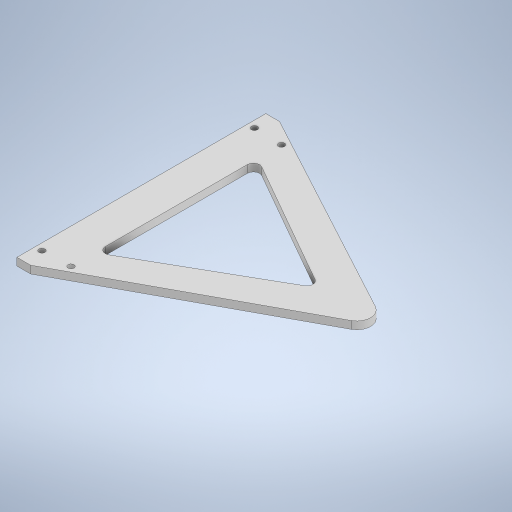
# Autodesk Inventor part: 17 nueva
Saved by Autodesk Inventor 2024.2 (Build 282272000, 272)
## iProperties
Created: 2024-10-10
Part Number: 17 nueva
Material: Generic
Document SubType Name: Modeling
Designer: Precisión-04
Density: 1 g/cm^3
Appearance: Default
Author: Precisión-04
Autodesk Inventor part; units mm, degrees
ref_plane "YZ Plane" through (0, 0, 0) normal (1, 0, 0) x (0, 1, 0)
ref_plane "XZ Plane" through (0, 0, 0) normal (0, 1, 0) x (-1, 0, 0)
ref_plane "XY Plane" through (0, 0, 0) normal (0, 0, 1) x (1, 0, 0)
sketch "Sketch1" plane through (0, 0, 0) normal (0, 1, 0) x (-1, 0, 0)
  line L0 (0, 0) -> (0, -164)
  line L1 (0, 0) -> (-9, 0)
  line L2 (0, -164) -> (-9, -164)
  line L3 (56.0828, -82) -> (-131.3763, -82) construction
  arc A0 (-146.3035, -74.0793) -> (-146.3035, -89.9207) centre (-142.03, -82) ccw
  line L4 (-110.9841, -85.4733) -> (-28.9841, -132.315)
  line L5 (-110.9833, -78.5263) -> (-28.9833, -31.7073)
  arc A1 (-23, -35.1809) -> (-28.9833, -31.7073) centre (-27, -35.1809) ccw
  arc A2 (-28.9841, -132.315) -> (-23, -128.8417) centre (-27, -128.8417) ccw
  line L6 (-23, -35.1809) -> (-23, -128.8417)
  line L7 (-146.3035, -89.9207) -> (-9, -164)
  line L8 (-9, 0) -> (-146.3035, -74.0793)
  arc A3 (-110.9833, -78.5263) -> (-110.9841, -85.4733) centre (-109, -82) ccw
  point P0 (0, -82)
  point P1 (-23, -82)
  point P2 (-75.5556, -35.9087)
  point P3 (-69.9833, -55.1168)
  point P4 (-75.5113, -128.1152)
  point P5 (-69.9841, -108.8941)
  dimension "d0" = 164
  dimension "d1" = 9
  dimension "d2" = 9
  dimension "d13" = 18
  dimension "d20" = 8
  dimension "d21" = 8
  dimension "d73" = 142.03
  dimension "d74" = 23
  dimension "d76" = 8
  dimension "d77" = 86
  dimension "d78" = 20
  dimension "d79" = 20
  constraints: 18 end point, 8 point on circle, 8 tangent, 7 point on line, 4 centre point, 3 horizontal, 3 midpoint, 2 vertical
  measures "d0" distance of L0.start L0.end
  measures "d1" distance of L0.start L1.end
  measures "d2" distance of L0.end L2.end
  measures "d13" diameter of A0
  measures "d20" diameter of A1
  measures "d21" diameter of A2
  measures "d73" distance from line of L0 A0.centre
  measures "d74" distance between parallel lines of L0 L6
  measures "d76" diameter of A3
  measures "d77" distance from line of L6 A3.centre
  measures "d78" distance of point (-75.556, -35.909) point (-69.983, -55.117)
  measures "d79" distance of point (-75.511, -128.115) point (-69.984, -108.894)
extrude "Extrusion1" add sketch "Sketch1" along normal blind 5
sketch "Sketch2" plane through (0, 5, 0) normal (0, 1, 0) x (1, 0, 0)
  line L0 (0, 164) -> (0, 0) projected
  line L1 (0, 82) -> (160.3523, 82) construction
  line L2 (4.5, 12) -> (4.5, 152) construction
  circle A0 centre (4.5, 12) radius 2
  circle A1 centre (4.5, 152) radius 2
  line L3 (23, 12.6666) -> (23, 144.7978) construction
  circle A2 centre (23, 12.6666) radius 2
  line L4 (23, 12.6666) -> (151.5071, 82) construction
  circle A3 centre (54.2428, 29.523) radius 2
  circle A4 centre (69.8202, 37.9275) radius 2
  line L5 (9, 0) -> (146.3035, 74.0793) projected
  circle A5 centre (85.3976, 46.3319) radius 2
  circle A6 centre (100.9749, 54.7364) radius 2
  circle A7 centre (116.5523, 63.1409) radius 2
  circle A8 centre (132.1297, 71.5453) radius 2
  circle A9 centre (38.6654, 21.1185) radius 2
  circle A10 centre (23, 151.3334) radius 2
  circle A11 centre (54.2428, 134.477) radius 2
  circle A12 centre (69.8202, 126.0725) radius 2
  circle A13 centre (85.3976, 117.6681) radius 2
  circle A14 centre (116.5523, 100.8591) radius 2
  circle A15 centre (132.1297, 92.4547) radius 2
  circle A16 centre (38.6654, 142.8815) radius 2
  point P0 (4.5, 82)
  point P1 (100.9749, 109.2636)
  dimension "d82" = 4
  dimension "d83" = 4
  dimension "d84" = 140
  dimension "d85" = 4.5
  dimension "d88" = 4
  dimension "d89" = 4
  dimension "d91" = 4
  dimension "d93" = 23
  dimension "d94" = 4.5
  dimension "d95" = 4.5
  dimension "d98" = 4
  dimension "d99" = 4
  dimension "d100" = 4
  dimension "d101" = 4
  dimension "d106" = 17.7
  dimension "d107" = 17.7
  dimension "d108" = 17.7
  dimension "d109" = 17.7
  dimension "d110" = 124
  dimension "d111" = 17.7
  dimension "d112" = 4
  dimension "d113" = 17.7
  constraints: 17 centre point, 8 symmetric about line, 6 end point, 3 coincident, 2 midpoint, 2 point on line, 2 vertical, 1 horizontal, 17 other
  measures "d82" diameter of A0
  measures "d83" diameter of A1
  measures "d84" distance of L2.start L2.end
  measures "d85" distance between parallel lines of L0 L2
  measures "d88" diameter of A2
  measures "d89" diameter of A3
  measures "d91" diameter of A4
  measures "d93" distance from line of L0 L3.start
  measures "d94" distance from line of L5 L3.start
  measures "d95" distance from line of L5 A3.centre
  measures "d98" diameter of A5
  measures "d99" diameter of A6
  measures "d100" diameter of A7
  measures "d101" diameter of A8
  measures "d106" distance of A7.centre A8.centre
  measures "d107" distance of A6.centre A7.centre
  measures "d108" distance of A6.centre A5.centre
  measures "d109" distance of A4.centre A5.centre
  measures "d110" distance of A8.centre A2.centre
  measures "d111" distance of A3.centre A4.centre
  measures "d112" diameter of A9
  measures "d113" distance of A3.centre A9.centre
hole "Hole2" at (4.5, 5, -12) at (23, 5, -12.6666) at (4.5, 5, -152) at (23, 5, -151.3334) direction (0, -1, 0) diameter 4 depth 10 tip angle 118
equation "\"d95\" = d94"
body "Solid1"
